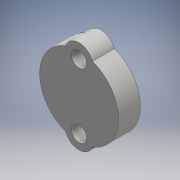
# Autodesk Inventor part: Ball Caster Spacer
Saved by Autodesk Inventor 2016 (Build 200138000, 138)
## iProperties
Created: 2017-03-04
Part Number: Ball Caster Spacer
Material: Generic
Document SubType Name: Modeling
Designer: Billy
Density: 1 g/cm^3
Appearance: Default
Author: Billy
Autodesk Inventor part; units mm, degrees
ref_plane "YZ Plane" through (0, 0, 0) normal (1, 0, 0) x (0, 1, 0)
ref_plane "XZ Plane" through (0, 0, 0) normal (0, 1, 0) x (-1, 0, 0)
ref_plane "XY Plane" through (0, 0, 0) normal (0, 0, 1) x (1, 0, 0)
sketch "Sketch1" plane through (0, 0, 0) normal (0, 1, 0) x (-1, 0, 0)
  circle A0 centre (0, 7.366) radius 1.75
  circle A1 centre (0, -7.366) radius 1.75
  arc A2 (3.0588, -8.4643) -> (3.0588, 8.4643) centre (0, 0) ccw
  arc A3 (-3.0588, 8.4643) -> (-3.0588, -8.4643) centre (0, 0) ccw
  arc A4 (3.0588, 8.4643) -> (-3.0588, 8.4643) centre (0, 7.366) ccw
  arc A5 (-3.0588, -8.4643) -> (3.0588, -8.4643) centre (0, -7.366) ccw
  point P0 (9, 0)
  constraints: 8 point on circle, 6 centre point
extrude "Extrusion1" add sketch "Sketch1" along normal blind 5
body "Solid1"
